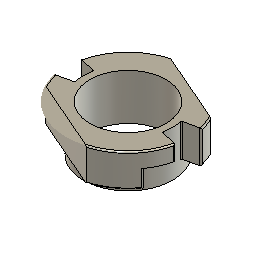
adaptateur_bouton_1of2 (Autodesk Fusion 360 design; units mm, degrees)
Autodesk Fusion 360 part; units mm, degrees
note: some values were not read from the file. Set by a fixed rule: which sketch regions a step uses.
sketch "Esquisse1" plane through (0, 0, 0) normal (0, 1, 0) x (1, 0, 0)
  circle A0 centre (0, 0) radius 11.9
  circle A1 centre (0, 0) radius 9.4
  circle A2 centre (0, 0) radius 6.8
  line L0 (-17.5, 1.45) -> (15, 1.45)
  line L1 (-17.5, -1.45) -> (15, -1.45)
  line L2 (15, -5.35) -> (-17.5, -5.35)
  line L3 (15, 5.35) -> (-17.5, 5.35)
  line L4 (7.729, 5.35) -> (-7.729, -5.35)
  line L5 (-7.729, 5.35) -> (7.729, -5.35)
  circle A3 centre (0, 0) radius 5.8
  line L6 (-17.5, 0) -> (15, 0)
  circle A4 centre (0, 0) radius 7.2
  line L7 (0, -15) -> (0, 15.3006)
  circle A5 centre (0, 0) radius 11.4
  line L8 (0, 0) -> (15.9266, -3.4786)
  line L9 (15.9266, -3.4786) -> (-17.8755, 3.9042)
  line L10 (0, 0) -> (18, 4)
  line L11 (18, 4) -> (-15.7974, -3.5105)
  line L12 (0, 0) -> (-18.1238, 7.8826)
  line L13 (-18.1238, 7.8826) -> (9.6293, -4.1881)
  line L14 (0, 0) -> (-5.6502, -12.991)
  line L15 (-5.6502, -12.991) -> (3.8538, 8.8607)
  line L16 (2.8717, 6.6025) -> (-20.8682, 16.9277)
  line L17 (-20.8682, 16.9277) -> (17.6302, 0.1836)
  line L18 (-2.8717, -6.6025) -> (-17.75, -0.1315)
  line L19 (-17.75, -0.1315) -> (11.0517, -12.6583)
  dimension "d6" = 23.8
  dimension "d20" = 3.9
  dimension "d21" = 3.9
  dimension "d51" = 1.45
  dimension "d52" = 1.45
  dimension "d60" = 18.8
  dimension "d61" = 13.6
  dimension "d62" = 0.4
  dimension "d70" = 2
  dimension "d75" = 90
  dimension "d76" = 90
  dimension "d77" = 90
  dimension "d82" = 22.37
  dimension "d85" = 11.185
  constraint coincident A0.centre A1.centre
  constraint horizontal L0
  constraint parallel L0 L1
  constraint horizontal L2
  constraint horizontal L3
  constraint coincident A1 L4.start
  constraint coincident L3 L4.start
  constraint coincident A1 L4.end
  constraint coincident L2 L4.end
  constraint coincident A1 L5.start
  constraint coincident L3 L5.start
  constraint coincident A1 L5.end
  constraint coincident L2 L5.end
  constraint concentric A0 A1
  constraint concentric A1 A2
  constraint horizontal L6
  constraint vertical L7
  constraint parallel L8 L9
  constraint parallel L10 L11
  constraint parallel L12 L13
  constraint parallel L14 L15
  constraint coincident L15 L16.start
  constraint coincident A4 L16.start
  constraint parallel L16 L17
  constraint coincident A4 L18.start
  constraint coincident L15 L18.start
  constraint parallel L18 L19
  measures "d6" diameter of A0
  measures "d20" distance of L1 L2
  measures "d21" distance of L0 L3
  measures "d51" distance of L0.end L6.end
  measures "d52" distance of L1 L6
  measures "d60" diameter of A1
  measures "d61" diameter of A2
  measures "d75" angle of L13 L15
  measures "d76" angle of L15 L17
  measures "d77" angle of L15 L18
  measures "d82" angle of L5 L9
  measures "d85" angle of L5 L12
extrude "Extrusion13" add sketch "Esquisse1" along normal blind 2 contours A0 L0 L6 A5 | A0 L1 L6 A5 | A0 L0 A5 L10 L11 | A0 L1 A5 L8 L9 | A1 L1 L6 A5 | A1 L0 L6 A5 | A0 A5 L10 L11 L17 | A1 L0 A5 L10 L11 | A0 L2 A5 L8 L9 | A1 L1 A5 L8 L9 | A1 L0 L6 A4 | A1 L1 L6 A4 | A0 L3 A5 L17 | A1 A5 L10 L11 L17 | A1 L0 A4 L10 L11 | A0 L2 A5 L19 | A1 L2 A5 L8 L9 | A1 L1 A4 L8 L9 | A0 L3 L7 A5 | A1 L3 A5 L17 | A1 L4 A4 L10 L11 L17 | A0 L7 A5 L19 | A1 L2 A5 L19 | A1 A4 L8 L9 L13 | A0 L7 A5 L16 L17 | A1 L3 L7 A5 | A1 L4 L17 | A0 L7 A5 L14 L15 | A1 L7 A5 L19 | A1 L5 A4 L13 | A1 L2 A4 L7 L19 | L2 L5 A4 | A0 L3 A5 L16 L17 | A1 L7 A5 L16 L17 | A1 L3 L15 L17 | L3 L4 L17 | L3 L4 A4 L17 | A0 L2 A5 L14 L15 | A1 L7 A5 L14 L15 | A1 L7 L19 | A0 L3 A5 L12 L13 | A1 L3 A5 L16 L17 | A1 L7 L16 L17 | A1 L7 L15 L16 L17 | L3 A4 L17 | A0 L2 A5 L18 L19 | A1 L2 A5 L14 L15 | A1 L7 L14 L15 L19 | A4 L7 L19 | A0 A5 L9 L12 L13 | A1 L3 A5 L12 L13 | A1 L3 A4 L7 L16 L17 | A4 L7 L16 L17 | A0 A5 L11 L18 L19 | A1 L2 A5 L18 L19 | A1 L2 L14 L15 L18 L19 | L2 A4 L18 L19 | A0 L0 A5 L9 | A1 A5 L9 L12 L13 | A1 L5 A4 L12 L13 | L3 L5 A4 | A0 L1 A5 L11 | A1 A5 L11 L18 L19 | L2 L4 L18 L19 | A1 L4 L18 L19 | L2 L4 A4 L18 L19 | A1 L1 L6 A4 | A1 L0 L6 A4 | A1 L0 A4 L9 | A1 A4 L9 L12 L13 | A0 L0 L6 A5 | A1 L0 A5 L9 | A0 L1 L6 A5 | A1 L1 A5 L11 | A1 L4 A4 L11 L18 L19 | A1 L1 A4 L11 | A1 L0 L6 A5 | A1 L1 L6 A5 makes body 1
extrude "Extrusion14" add sketch "Esquisse1" along normal blind 5 separate body contours A1 L0 L6 A4 | A1 L1 L6 A4 | A1 L0 A4 L10 L11 | A1 L1 A4 L8 L9 | A2 L1 L6 A4 | A2 L0 L6 A4 | A1 L4 A4 L10 L11 L17 | A2 L0 A4 L10 L11 | A1 A4 L8 L9 L13 | L1 A4 L8 L9 | A1 L4 L17 | A2 L4 A4 L10 L11 | A1 L5 A4 L13 | A1 L2 A4 L7 L19 | L2 L5 A4 | A2 A4 L8 L9 L13 | A1 L3 L15 L17 | L3 L4 L17 | L3 L4 A4 L17 | A2 L3 L4 A4 | A1 L7 L19 | A2 L2 A4 L7 | A2 L2 L5 A4 | A2 L5 A4 L13 | A1 L7 L16 L17 | A1 L7 L15 L16 L17 | L3 A4 L17 | A2 L3 A4 L15 | A1 L7 L14 L15 L19 | A4 L7 L19 | A2 A4 L7 L14 L15 | A1 L3 A4 L7 L16 L17 | A4 L7 L16 L17 | A2 A4 L7 L15 | A1 L2 L14 L15 L18 L19 | L2 A4 L18 L19 | A2 L2 A4 L14 L15 | A2 L0 L6 A4 | A2 L1 L6 A4 | A2 A4 L9 L12 L13 | L0 A4 L9 | A1 L5 A4 L12 L13 | L3 L5 A4 | A2 L3 A4 L7 | L2 L4 L18 L19 | A1 L4 L18 L19 | A2 L2 L4 A4 | L2 L4 A4 L18 L19 | A2 L4 A4 L11 | A2 L3 L5 A4 | A2 L5 A4 L12 L13 | A2 L1 A4 L11 | A1 L1 L6 A4 | A1 L0 L6 A4 | A1 L0 A4 L9 | A1 A4 L9 L12 L13 | A1 L4 A4 L11 L18 L19 | A1 L1 A4 L11 makes body 2
move_body "Déplacer2" bodies 1 to x (1, 0, 0) y (0, 1, 0) z (0, 0, 1) at (0, -5, 0)
extrude "Extrusion15" cut sketch "Esquisse1" along normal blind 2.7 contours A1 L0 L6 A4 | A1 L1 L6 A4 | A1 L1 A4 L8 L9 | A2 L1 L6 A4 | A2 L0 L6 A4 | A2 L0 A4 L10 L11 | A1 A4 L8 L9 L13 | A1 L5 A4 L13 | A2 A4 L8 L9 L13 | A2 L5 A4 L13 | A2 L0 L6 A4 | A2 L1 L6 A4 | A2 A4 L9 L12 L13 | A1 L5 A4 L12 L13 | A2 L5 A4 L12 L13 | A2 L1 A4 L11 | A1 L1 L6 A4 | A1 L0 L6 A4 | A1 L0 A4 L9 | A1 A4 L9 L12 L13 | A1 L1 A4 L11 bodies 2
extrude "Extrusion16" cut sketch "Esquisse1" along normal blind 23.8 contours A1 L0 L6 A4 | A1 L1 L6 A4 | A1 L0 A4 L10 L11 | A1 L1 A4 L8 L9 | A2 L1 L6 A4 | A2 L0 L6 A4 | A2 L0 A4 L10 L11 | L1 A4 L8 L9 | A2 L0 L6 A4 | A2 L1 L6 A4 | L0 A4 L9 | A2 L1 A4 L11 | A1 L1 L6 A4 | A1 L0 L6 A4 | A1 L0 A4 L9 | A1 L1 A4 L11 bodies 2 makes body 3 at (7.1063, 2.5667, 6.1531)
extrude "Extrusion17" add sketch "Esquisse1" along normal blind 5 contours A2 L0 A3 L6 L10 L11 | A2 A3 L6 L8 L9 | A2 L0 L10 L11 | A2 L1 A3 L13 | L1 A3 L8 L9 | A2 L0 L4 A3 L10 L11 | L0 A3 L10 L11 | A2 L5 A3 L13 | A2 L3 L4 A3 L15 | A2 L2 L5 A3 | A2 L2 A3 L7 | A2 A3 L6 L9 | A2 L1 A3 L6 L11 | L0 A3 L9 | L1 A3 L11 | A2 L3 L15 | A2 L2 A3 L7 L14 L15 | A2 L1 L4 A3 L11 | A2 L2 L4 A3 L14 L15 | A2 L5 A3 L12 L13 | A2 L3 L5 A3 | A2 L0 A3 L12 L13 | A2 L1 L11 | L2 A3 L14 L15 | L3 A3 L15 | A2 L3 A3 L7 L15 | A2 L2 L14 L15 | A2 L3 A3 L7 bodies 2 3
extrude "Extrusion18" add sketch "Esquisse1" against normal blind 2 contours A2 L0 A3 L6 L10 L11 | A2 A3 L6 L8 L9 | A2 L0 L10 L11 | A2 L1 A3 L13 | L1 A3 L8 L9 | A2 L0 L4 A3 L10 L11 | L0 A3 L10 L11 | A2 L5 A3 L13 | A2 L3 L4 A3 L15 | A2 L2 L5 A3 | A2 L2 A3 L7 | A2 A3 L6 L9 | A2 L1 A3 L6 L11 | L0 A3 L9 | L1 A3 L11 | A2 L3 L15 | A2 L2 A3 L7 L14 L15 | A2 L1 L4 A3 L11 | A2 L2 L4 A3 L14 L15 | A2 L5 A3 L12 L13 | A2 L3 L5 A3 | A2 L0 A3 L12 L13 | A2 L1 L11 | L2 A3 L14 L15 | L3 A3 L15 | A2 L3 A3 L7 L15 | A2 L2 L14 L15 | A2 L3 A3 L7 bodies 2
extrude "Extrusion23" cut sketch "Esquisse1" along normal blind 5 contours A1 L4 L17 | A1 L3 L15 L17 | L3 L4 L17 | A1 L7 L19 | A1 L7 L16 L17 | A1 L7 L15 L16 L17 | A1 L7 L14 L15 L19 | A1 L2 L14 L15 L18 L19 | L2 L4 L18 L19 | A1 L4 L18 L19 bodies 2
fillet "Congé2" radius 0.2 24 edges at (-7.729, 1.35, -5.35) (7.729, 1.35, 5.35) (9.1835, 3.85, 2.0058) (-9.1835, 3.85, -2.0058) (-6.6434, 3.85, -1.451) (-5.5912, 1.35, -3.8702) (-5.5126, 0, -7.6139) (-6.8849, 5, -6.3999) (-9.1762, 2.5, 2.0391) (-8.8604, 5, 3.139) (-8.8604, 0, 3.139) (5.5126, 0, 7.6139) (-6.6381, 2.5, 1.4751) (8.8604, 0, -3.139) (8.8604, 5, -3.139) (9.1762, 2.5, -2.0391) (6.6381, 2.5, -1.4751) (6.8849, 5, 6.3999) (9.1835, 3.85, 2.0058) (-9.1835, 3.85, -2.0058) (-7.729, 1.35, -5.35) (7.729, 1.35, 5.35) (5.5912, 1.35, 3.8702) (6.6434, 3.85, 1.451) on bodies 2
hidden bodies 1
equation "dia_ext_tube_bouton = 23.8 mm"
equation "dia_int_tube_bouton = 19 mm"
equation "largeur_ergot = 2.5 mm"
equation "epaissur_ergot = 2.5 mm"
equation "jeu = 0.2 mm"
equation "d6 = dia_ext_tube_bouton"
equation "epaisseur_tube_support = 2 mm"
equation "d20 = largeur_ergot + jeu * 2 + 1 mm"
equation "d21 = d20"
equation "d42 = -epaisseur_tube_jonction"
equation "epaisseur_tube_jonction = 1 mm"
equation "d44 = epaisseur_collerette"
equation "profondeur_ergot = 2.5 mm"
equation "d47 = epaissur_ergot * 2"
equation "d49 = epaissur_ergot + jeu"
equation "d51 = largeur_ergot / 2 + jeu"
equation "d52 = d51"
equation "d53 = dia_ext_tube_bouton"
equation "d55 = d47"
equation "epaisseur_collerette = 2 mm"
equation "d58 = -epaisseur_collerette"
equation "d60 = dia_int_tube_bouton - jeu"
equation "d61 = dia_int_tube_bouton - profondeur_ergot * 2 - jeu * 2"
equation "d62 = jeu * 2"
equation "largeur_doigt = 4 mm"
equation "d66 = largeur_doigt"
equation "d70 = largeur_doigt / 2"
equation "d85 = d82 / 2"
equation "d88 = d47"
